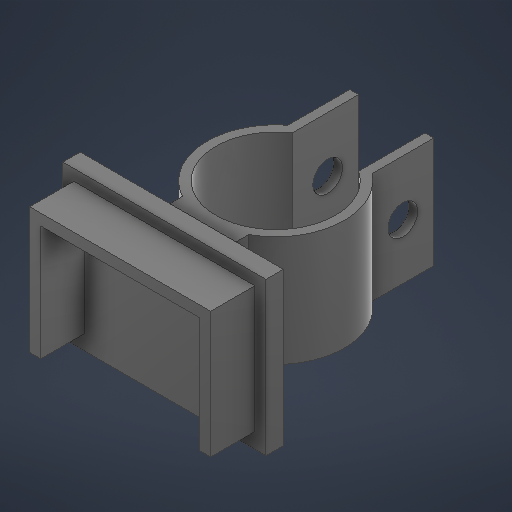
# Autodesk Inventor part: microphone_casing_back
Saved by Autodesk Inventor 2026 (Build 300175050, 175E)
## iProperties
Created: 2025-06-09
Part Number: microphone_casing_back
Material: Generic
Document SubType Name: Modeling
Designer: satom
Density: 1 g/cm^3
Appearance: Default
Author: satom
Autodesk Inventor part; units mm, degrees
ref_plane "YZ Plane" through (0, 0, 0) normal (1, 0, 0) x (0, 1, 0)
ref_plane "XZ Plane" through (0, 0, 0) normal (0, 1, 0) x (-1, 0, 0)
ref_plane "XY Plane" through (0, 0, 0) normal (0, 0, 1) x (1, 0, 0)
sketch "Sketch1" plane through (0, 0, 0) normal (0, 0, 1) x (1, 0, 0)
  line L0 (0, 0) -> (23.33, 0)
  line L1 (23.33, 0) -> (23.33, 17.54)
  line L2 (23.33, 17.54) -> (0, 17.54)
  line L3 (0, 17.54) -> (0, 0)
  dimension "d0" = 23.33
  dimension "d1" = 17.54
  constraints: 8 end point, 2 parallel, 1 horizontal, 1 perpendicular
  measures "d0" distance of L1.end L2.end
  measures "d1" distance of L0.end L1.end
extrude "Extrusion1" add sketch "Sketch1" along normal blind 2
sketch "Sketch2" plane through (0, 0, 2) normal (0, 0, 1) x (1, 0, 0)
  line L0 (22.06, 1.778) -> (22.06, 16.27)
  line L1 (22.06, 16.27) -> (1.27, 16.27)
  line L2 (1.27, 16.27) -> (1.27, 1.778)
  line L3 (0, 17.54) -> (0, 0) projected
  line L4 (23.33, 0) -> (23.33, 17.54) projected
  line L5 (23.33, 17.54) -> (0, 17.54) projected
  line L6 (0, 0) -> (23.33, 0) projected
  line L7 (2.54, 1.778) -> (2.54, 15)
  line L8 (2.54, 15) -> (20.79, 15)
  line L9 (20.79, 15) -> (20.79, 1.778)
  line L10 (1.27, 1.778) -> (2.54, 1.778)
  line L11 (20.79, 1.778) -> (22.06, 1.778)
  dimension "d4" = 1.27
  dimension "d5" = 1.27
  dimension "d7" = 1.778
  dimension "d8" = 1.778
  dimension "d9" = 1.27
  dimension "d10" = 1.27
  constraints: 16 end point, 3 equal length, 1 horizontal, 2 other
  measures "d4" distance between parallel lines of L3 L2
  measures "d5" distance between parallel lines of L4 L0
  measures "d7" distance from line of L6 L0.start
  measures "d8" distance from line of L6 L2.end
  measures "d9" distance between parallel lines of L5 L1
  measures "d10" distance between parallel lines of L2 L7
extrude "Extrusion2" add sketch "Sketch2" along normal blind 5.08 contours L11 L9 L8 L7 L10 L2 L1 L0
sketch "Sketch3" plane through (0, 0, 0) normal (0, 0, -1) x (-1, 0, 0)
  line L0 (-23.33, 0) -> (-23.33, 17.54) construction
  line L1 (-23.33, 8.77) -> (0, 8.77) construction
  line L2 (0, 17.54) -> (0, 0) construction
  line L3 (-23.33, 17.54) -> (0, 17.54) construction
  line L4 (-11.665, 17.54) -> (-11.665, 0) construction
  line L5 (0, 0) -> (-23.33, 0) construction
  line L6 (-15.475, 2.42) -> (-7.855, 2.42)
  line L7 (-7.855, 2.42) -> (-7.855, 15.12)
  line L8 (-7.855, 15.12) -> (-15.475, 15.12)
  line L9 (-15.475, 15.12) -> (-15.475, 2.42)
  line L10 (-15.475, 2.42) -> (-7.855, 15.12) construction
  line L11 (-7.855, 2.42) -> (-15.475, 15.12) construction
  point P0 (-11.665, 8.77)
  dimension "d13" = 12.7
  dimension "d14" = 7.62
  constraints: 16 end point, 7 midpoint, 2 horizontal, 2 parallel, 1 perpendicular, 1 vertical
  measures "d13" distance of L8.end L6.start
  measures "d14" distance of L7.end L8.end
extrude "Extrusion3" add sketch "Sketch3" along normal blind 5.08
sketch "Sketch4" plane through (7.855, 15.12, 0) normal (0, 1, 0) x (1, 0, 0)
  line L0 (7.62, 5.08) -> (0, 5.08) construction
  line L1 (3.81, 5.08) -> (3.81, 10.7823) construction
  circle A0 centre (3.81, 10.7823) radius 6.858
  point P0 (-7.855, 0)
  dimension "d17" = 5.7023
  constraints: 2 end point, 1 coincident, 1 midpoint, 1 vertical, 3 other
  measures "d17" distance of L1.start L1.end
extrude "Extrusion4" cut sketch "Sketch4" against normal through all
sketch "Sketch5" plane through (7.855, 15.12, 0) normal (0, 1, 0) x (1, 0, 0)
  arc A0 (0, 5.08) -> (7.62, 5.08) centre (3.81, 10.7823) ccw projected
  line L0 (3.81, 3.9243) -> (3.81, 2.9083) construction
  arc A1 (-1.016, 17.004) -> (8.636, 17.004) centre (3.81, 10.7823) ccw
  line L1 (0, 5.08) -> (0, 21.0009) construction
  line L2 (7.62, 5.08) -> (7.62, 21.4272) construction
  arc A2 (7.62, 5.08) -> (7.62, 16.4846) centre (3.81, 10.7823) ccw
  arc A3 (0, 16.4846) -> (3.81, 3.9243) centre (3.81, 10.7823) ccw
  line L3 (7.62, 16.4846) -> (8.636, 16.4846) construction
  line L4 (0, 16.4846) -> (-1.016, 16.4846) construction
  line L5 (8.636, 17.004) -> (8.636, 24.1225)
  line L6 (-1.016, 17.004) -> (-1.016, 24.1225)
  line L7 (8.636, 24.1225) -> (7.62, 24.1225)
  line L8 (7.62, 24.1225) -> (7.62, 16.4846)
  line L9 (-1.016, 24.1225) -> (0, 24.1225)
  line L10 (0, 24.1225) -> (0, 16.4846)
  point P0 (-7.855, 0)
  dimension "d20" = 1.016
  dimension "d21" = 1.016
  dimension "d22" = 1.016
  dimension "d23" = 7.1185
  dimension "d24" = 7.1185
  constraints: 22 end point, 9 point on circle, 5 vertical, 3 centre point, 3 horizontal, 3 point on line, 1 coincident, 1 collinear, 1 perpendicular
  measures "d20" distance of L0.start L0.end
  measures "d21" distance of L3.start L3.end
  measures "d22" distance of L4.start L4.end
  measures "d23" distance of L5.start L5.end
  measures "d24" distance of L6.start L6.end
extrude "Extrusion5" add sketch "Sketch5" against normal blind 12.7
sketch "Sketch6" plane through (6.839, 15.12, -24.1225) normal (-1, 0, 0) x (0, 0, 1)
  line L0 (0, 0) -> (0, -12.7) construction
  line L1 (7.1185, -12.7) -> (20.2311, -12.7) construction
  line L2 (0, 0) -> (7.1185, -12.7) construction
  line L3 (20.2311, 0) -> (7.1185, 0) construction
  line L4 (7.1185, -12.7) -> (0, -12.7) construction
  line L5 (7.1185, 0) -> (0, -12.7) construction
  circle A0 centre (3.5593, -6.35) radius 1.7
  point P0 (24.1225, -15.12)
  dimension "d27" = 3.4
  constraints: 4 end point, 2 midpoint, 1 centre point
  measures "d27" diameter of A0
extrude "Extrusion6" cut sketch "Sketch6" against normal through all
equation "\"d5\" = d4"
equation "\"d8\" = d7"
equation "\"d9\" = d4"
equation "\"d24\" = d23"
equation "\"d27\" = m3_clearance"
equation "\"m3_heat_set_insert\" = 4"
equation "\"m3_clearance\" = 3.4"
equation "\"m3_heat_set_depth\" = 7"
equation "\"robot_diameter\" = 354"
equation "\"hardboard_thickness\" = 5"
equation "\"motor_centerline_height\" = 13"
body "Solid1"
